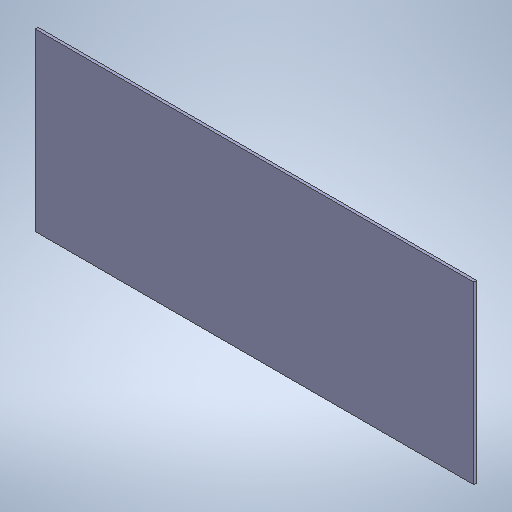
# Autodesk Inventor part: RoofCover
Saved by Autodesk Inventor 2026.2 (Build 302298010, 298A)
## iProperties
Created: 2026-03-20
Part Number: RoofCover
Material: Ogólny
Document SubType Name: Modeling
Designer: Patryk
Density: 1 g/cm^3
Appearance: Domyślna
Author: Patryk
Autodesk Inventor part; units mm, degrees
ref_plane "YZ Plane" through (0, 0, 0) normal (1, 0, 0) x (0, 1, 0)
ref_plane "XZ Plane" through (0, 0, 0) normal (0, 1, 0) x (-1, 0, 0)
ref_plane "XY Plane" through (0, 0, 0) normal (0, 0, 1) x (1, 0, 0)
sketch "Szkic1" plane through (0, 0, 0) normal (0, 0, 1) x (1, 0, 0)
  line L0 (150, -60) -> (-150, -60)
  line L1 (-150, -60) -> (-150, 60)
  line L2 (-150, 60) -> (150, 60)
  line L3 (150, 60) -> (150, -60)
  line L4 (150, -60) -> (-150, 60) construction
  line L5 (-150, -60) -> (150, 60) construction
  point P0 (0, 0)
  dimension "d0" = 300
  dimension "d1" = 120
  constraints: 12 end point, 2 midpoint, 2 parallel, 1 horizontal, 1 perpendicular
  measures "d0" distance of L1.end L2.end
  measures "d1" distance of L2.end L0.start
extrude "Wyciągnięcie proste1" add sketch "Szkic1" along normal mid plane 2
